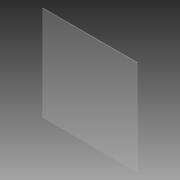
# Autodesk Inventor part: splash guard
Saved by Autodesk Inventor 2011 (Build 150239000, 239)
## iProperties
Created: 2014-01-03
Part Number: splash guard
Document SubType Name: Modeling
Designer: Devon
Density: 1 g/cm^3
Author: Devon
Autodesk Inventor part; units mm, degrees
ref_plane "YZ Plane" through (0, 0, 0) normal (1, 0, 0) x (0, 1, 0)
ref_plane "XZ Plane" through (0, 0, 0) normal (0, 1, 0) x (-1, 0, 0)
ref_plane "XY Plane" through (0, 0, 0) normal (0, 0, 1) x (1, 0, 0)
sketch "Sketch1" plane through (0, 0, 0) normal (0, 0, 1) x (1, 0, 0)
  line L0 (0, 0) -> (634.1872, 0)
  line L1 (634.1872, 0) -> (634.1872, 634.1872)
  line L2 (634.1872, 634.1872) -> (0, 634.1872)
  line L3 (0, 634.1872) -> (0, 0)
  dimension "d0" = 634.1872
  dimension "d1" = 634.1872
  constraints: 8 end point, 2 parallel, 1 horizontal, 1 perpendicular
  measures "d0" distance of L2.end L1.end
  measures "d1" distance of L1.end L0.end
extrude "Extrusion1" add sketch "Sketch1" along normal blind 6.35
body "Solid1"
